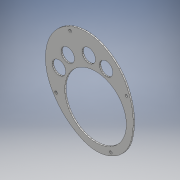
# Autodesk Inventor part: Mano-licar
Saved by Autodesk Inventor 2018 (Build 220112000, 112)
## iProperties
Created: 2019-01-30
Part Number: Mano-licar
Material: Generic
Document SubType Name: Modeling
Designer: Estudiante
Density: 1 g/cm^3
Appearance: Default
Author: Estudiante
Autodesk Inventor part; units mm, degrees
ref_plane "YZ Plane" through (0, 0, 0) normal (1, 0, 0) x (0, 1, 0)
ref_plane "XZ Plane" through (0, 0, 0) normal (0, 1, 0) x (-1, 0, 0)
ref_plane "XY Plane" through (0, 0, 0) normal (0, 0, 1) x (1, 0, 0)
sketch "Sketch1" plane through (0, 0, 0) normal (0, 1, 0) x (-1, 0, 0)
  line L0 (39.5804, 21.3013) -> (36.969, 22.6578)
  line L1 (51.1808, 16.6745) -> (52.2099, 17.5662)
  line L2 (53.4414, 18.1472) -> (52.2099, 17.5662)
  line L3 (54.784, 18.3744) -> (53.4414, 18.1472)
  line L4 (56.1381, 18.231) -> (54.784, 18.3744)
  line L5 (57.4032, 17.7275) -> (56.1381, 18.231)
  line L6 (58.4857, 16.9014) -> (57.4032, 17.7275)
  line L7 (59.3051, 15.8139) -> (58.4857, 16.9014)
  line L8 (59.8007, 14.5456) -> (59.3051, 15.8139)
  line L9 (59.9357, 13.1907) -> (59.8007, 14.5456)
  line L10 (59.7002, 11.8495) -> (59.9357, 13.1907)
  line L11 (59.1116, 10.6216) -> (59.7002, 11.8495)
  line L12 (58.2135, 9.5981) -> (59.1116, 10.6216)
  line L13 (57.0726, 8.8548) -> (58.2135, 9.5981)
  line L14 (55.7735, 8.4469) -> (57.0726, 8.8548)
  line L15 (54.4125, 8.4047) -> (55.7735, 8.4469)
  line L16 (53.0905, 8.7311) -> (54.4125, 8.4047)
  line L17 (51.9057, 9.4022) -> (53.0905, 8.7311)
  line L18 (50.9458, 10.368) -> (51.9057, 9.4022)
  line L19 (50.2822, 11.557) -> (50.9458, 10.368)
  line L20 (49.9639, 12.8809) -> (50.2822, 11.557)
  line L21 (50.0146, 14.2417) -> (49.9639, 12.8809)
  line L22 (50.4305, 15.5382) -> (50.0146, 14.2417)
  line L23 (51.1808, 16.6745) -> (50.4305, 15.5382)
  line L24 (59.8717, 33.0327) -> (61.5031, 30.232)
  line L25 (57.9468, 35.6404) -> (59.8717, 33.0327)
  line L26 (55.751, 38.0245) -> (57.9468, 35.6404)
  line L27 (53.3101, 40.157) -> (55.751, 38.0245)
  line L28 (50.6528, 42.0128) -> (53.3101, 40.157)
  line L29 (47.8103, 43.5703) -> (50.6528, 42.0128)
  line L30 (44.816, 44.8109) -> (47.8103, 43.5703)
  line L31 (41.705, 45.7203) -> (44.816, 44.8109)
  line L32 (38.5138, 46.2877) -> (41.705, 45.7203)
  line L33 (35.28, 46.5065) -> (38.5138, 46.2877)
  line L34 (32.0415, 46.374) -> (35.28, 46.5065)
  line L35 (28.8364, 45.8919) -> (32.0415, 46.374)
  line L36 (25.7022, 45.0658) -> (28.8364, 45.8919)
  line L37 (25.7022, 45.0658) -> (22.2386, 43.6878)
  line L38 (18.9322, 41.9665) -> (22.2386, 43.6878)
  line L39 (15.8169, 39.9196) -> (18.9322, 41.9665)
  line L40 (12.9246, 37.568) -> (15.8169, 39.9196)
  line L41 (10.285, 34.9359) -> (12.9246, 37.568)
  line L42 (7.9252, 32.0504) -> (10.285, 34.9359)
  line L43 (5.8694, 28.9409) -> (7.9252, 32.0504)
  line L44 (4.1387, 25.6393) -> (5.8694, 28.9409)
  line L45 (2.7509, 22.1797) -> (4.1387, 25.6393)
  line L46 (2.7509, 22.1797) -> (1.5483, 18.5508)
  line L47 (0.6396, 14.8374) -> (1.5483, 18.5508)
  line L48 (0.0306, 11.0633) -> (0.6396, 14.8374)
  line L49 (-0.275, 7.2526) -> (0.0306, 11.0633)
  line L50 (-0.275, 3.4296) -> (-0.275, 7.2526)
  line L51 (0.0306, -0.3811) -> (-0.275, 3.4296)
  line L52 (0.6396, -4.1552) -> (0.0306, -0.3811)
  line L53 (1.5483, -7.8686) -> (0.6396, -4.1552)
  line L54 (1.5483, -7.8686) -> (2.5978, -10.8174)
  line L55 (4.0034, -13.6141) -> (2.5978, -10.8174)
  line L56 (5.7437, -16.2157) -> (4.0034, -13.6141)
  line L57 (7.7921, -18.5824) -> (5.7437, -16.2157)
  line L58 (10.117, -20.678) -> (7.7921, -18.5824)
  line L59 (12.6831, -22.4704) -> (10.117, -20.678)
  line L60 (15.4508, -23.9321) -> (12.6831, -22.4704)
  line L61 (15.4508, -23.9321) -> (18.3237, -25.1744)
  line L62 (21.3281, -26.0524) -> (18.3237, -25.1744)
  line L63 (24.4179, -26.5526) -> (21.3281, -26.0524)
  line L64 (27.5458, -26.6672) -> (24.4179, -26.5526)
  line L65 (30.664, -26.3947) -> (27.5458, -26.6672)
  line L66 (33.7246, -25.7391) -> (30.664, -26.3947)
  line L67 (36.6808, -24.7105) -> (33.7246, -25.7391)
  line L68 (36.6808, -24.7105) -> (40.1448, -23.0933)
  line L69 (43.4686, -21.2046) -> (40.1448, -23.0933)
  line L70 (46.6308, -19.0562) -> (43.4686, -21.2046)
  line L71 (49.6112, -16.662) -> (46.6308, -19.0562)
  line L72 (52.3907, -14.0373) -> (49.6112, -16.662)
  line L73 (54.9516, -11.1989) -> (52.3907, -14.0373)
  line L74 (57.2775, -8.1648) -> (54.9516, -11.1989)
  line L75 (59.3535, -4.9547) -> (57.2775, -8.1648)
  line L76 (59.3535, -4.9547) -> (61.1815, -1.706)
  line L77 (62.6715, 1.7109) -> (61.1815, -1.706)
  line L78 (63.8082, 5.261) -> (62.6715, 1.7109)
  line L79 (64.5799, 8.9078) -> (63.8082, 5.261)
  line L80 (64.9788, 12.6141) -> (64.5799, 8.9078)
  line L81 (65.0008, 16.3416) -> (64.9788, 12.6141)
  line L82 (64.6455, 20.0523) -> (65.0008, 16.3416)
  line L83 (63.9167, 23.708) -> (64.6455, 20.0523)
  line L84 (62.8219, 27.2712) -> (63.9167, 23.708)
  line L85 (61.5031, 30.232) -> (62.8219, 27.2712)
  line L86 (49.2473, 19.8424) -> (50.5464, 20.2503)
  line L87 (47.8862, 19.8002) -> (49.2473, 19.8424)
  line L88 (46.5643, 20.1267) -> (47.8862, 19.8002)
  line L89 (45.3795, 20.7977) -> (46.5643, 20.1267)
  line L90 (44.4196, 21.7635) -> (45.3795, 20.7977)
  line L91 (43.7559, 22.9525) -> (44.4196, 21.7635)
  line L92 (43.4376, 24.2764) -> (43.7559, 22.9525)
  line L93 (43.4883, 25.6372) -> (43.4376, 24.2764)
  line L94 (43.9043, 26.9337) -> (43.4883, 25.6372)
  line L95 (44.6546, 28.07) -> (43.9043, 26.9337)
  line L96 (44.6546, 28.07) -> (45.6837, 28.9617)
  line L97 (46.9152, 29.5427) -> (45.6837, 28.9617)
  line L98 (48.2578, 29.7699) -> (46.9152, 29.5427)
  line L99 (49.6118, 29.6265) -> (48.2578, 29.7699)
  line L100 (50.877, 29.123) -> (49.6118, 29.6265)
  line L101 (51.9594, 28.2969) -> (50.877, 29.123)
  line L102 (52.7788, 27.2094) -> (51.9594, 28.2969)
  line L103 (53.2745, 25.9411) -> (52.7788, 27.2094)
  line L104 (53.4095, 24.5862) -> (53.2745, 25.9411)
  line L105 (53.174, 23.245) -> (53.4095, 24.5862)
  line L106 (52.5854, 22.0172) -> (53.174, 23.245)
  line L107 (51.6873, 20.9936) -> (52.5854, 22.0172)
  line L108 (50.5464, 20.2503) -> (51.6873, 20.9936)
  line L109 (45.6686, 41.0487) -> (45.8931, 40.5319)
  line L110 (45.6686, 41.0487) -> (45.7592, 41.6049)
  line L111 (45.7592, 41.6049) -> (46.136, 42.0238)
  line L112 (46.136, 42.0238) -> (46.6795, 42.1724)
  line L113 (47.2171, 42.0036) -> (46.6795, 42.1724)
  line L114 (47.5781, 41.571) -> (47.2171, 42.0036)
  line L115 (47.6479, 41.0119) -> (47.5781, 41.571)
  line L116 (47.4044, 40.5038) -> (47.6479, 41.0119)
  line L117 (46.9247, 40.208) -> (47.4044, 40.5038)
  line L118 (46.3614, 40.2185) -> (46.9247, 40.208)
  line L119 (45.8931, 40.5319) -> (46.3614, 40.2185)
  line L120 (36.9503, 29.5123) -> (37.539, 30.7402)
  line L121 (36.0523, 28.4888) -> (36.9503, 29.5123)
  line L122 (34.9114, 27.7455) -> (36.0523, 28.4888)
  line L123 (33.6122, 27.3376) -> (34.9114, 27.7455)
  line L124 (32.2512, 27.2953) -> (33.6122, 27.3376)
  line L125 (30.9293, 27.6218) -> (32.2512, 27.2953)
  line L126 (29.7444, 28.2929) -> (30.9293, 27.6218)
  line L127 (28.7846, 29.2587) -> (29.7444, 28.2929)
  line L128 (28.1209, 30.4477) -> (28.7846, 29.2587)
  line L129 (27.8026, 31.7716) -> (28.1209, 30.4477)
  line L130 (27.8533, 33.1323) -> (27.8026, 31.7716)
  line L131 (28.2692, 34.4289) -> (27.8533, 33.1323)
  line L132 (29.0196, 35.5652) -> (28.2692, 34.4289)
  line L133 (29.0196, 35.5652) -> (30.0486, 36.4569)
  line L134 (31.2801, 37.0379) -> (30.0486, 36.4569)
  line L135 (32.6227, 37.2651) -> (31.2801, 37.0379)
  line L136 (33.9768, 37.1217) -> (32.6227, 37.2651)
  line L137 (35.242, 36.6182) -> (33.9768, 37.1217)
  line L138 (36.3244, 35.7921) -> (35.242, 36.6182)
  line L139 (37.1438, 34.7046) -> (36.3244, 35.7921)
  line L140 (37.6394, 33.4363) -> (37.1438, 34.7046)
  line L141 (37.7745, 32.0813) -> (37.6394, 33.4363)
  line L142 (37.539, 30.7402) -> (37.7745, 32.0813)
  line L143 (19.8181, -19.9229) -> (22.6407, -20.7551)
  line L144 (17.1252, -18.7365) -> (19.8181, -19.9229)
  line L145 (14.6061, -17.2156) -> (17.1252, -18.7365)
  line L146 (12.3022, -15.385) -> (14.6061, -17.2156)
  line L147 (10.2513, -13.2748) -> (12.3022, -15.385)
  line L148 (8.4871, -10.9196) -> (10.2513, -13.2748)
  line L149 (7.0385, -8.3582) -> (8.4871, -10.9196)
  line L150 (5.9294, -5.6326) -> (7.0385, -8.3582)
  line L151 (5.1779, -2.7875) -> (5.9294, -5.6326)
  line L152 (4.7964, 0.1303) -> (5.1779, -2.7875)
  line L153 (4.7912, 3.073) -> (4.7964, 0.1303)
  line L154 (5.1623, 5.9921) -> (4.7912, 3.073)
  line L155 (5.9036, 8.8399) -> (5.1623, 5.9921)
  line L156 (5.9036, 8.8399) -> (7.003, 11.5694)
  line L157 (7.003, 11.5694) -> (8.4425, 14.136)
  line L158 (8.4425, 14.136) -> (10.1983, 16.4974)
  line L159 (12.2417, 18.6149) -> (10.1983, 16.4974)
  line L160 (14.5391, 20.4537) -> (12.2417, 18.6149)
  line L161 (17.0527, 21.9836) -> (14.5391, 20.4537)
  line L162 (19.7414, 23.1795) -> (17.0527, 21.9836)
  line L163 (22.561, 24.0218) -> (19.7414, 23.1795)
  line L164 (25.465, 24.4966) -> (22.561, 24.0218)
  line L165 (28.406, 24.5962) -> (25.465, 24.4966)
  line L166 (31.3356, 24.3188) -> (28.406, 24.5962)
  line L167 (34.2056, 23.6692) -> (31.3356, 24.3188)
  line L168 (36.969, 22.6578) -> (34.2056, 23.6692)
  line L169 (39.5804, 21.3013) -> (36.969, 22.6578)
  line L170 (41.9968, 19.6221) -> (39.5804, 21.3013)
  line L171 (44.1787, 17.6476) -> (41.9968, 19.6221)
  line L172 (46.0902, 15.4104) -> (44.1787, 17.6476)
  line L173 (47.6999, 12.947) -> (46.0902, 15.4104)
  line L174 (48.9814, 10.2981) -> (47.6999, 12.947)
  line L175 (49.9137, 7.507) -> (48.9814, 10.2981)
  line L176 (50.4813, 4.6196) -> (49.9137, 7.507)
  line L177 (50.6751, 1.6833) -> (50.4813, 4.6196)
  line L178 (50.4918, -1.2536) -> (50.6751, 1.6833)
  line L179 (49.9344, -4.143) -> (50.4918, -1.2536)
  line L180 (49.0121, -6.9374) -> (49.9344, -4.143)
  line L181 (47.7401, -9.5909) -> (49.0121, -6.9374)
  line L182 (46.1391, -12.0599) -> (47.7401, -9.5909)
  line L183 (44.2356, -14.304) -> (46.1391, -12.0599)
  line L184 (42.0608, -16.2862) -> (44.2356, -14.304)
  line L185 (39.6503, -17.9741) -> (42.0608, -16.2862)
  line L186 (37.0438, -19.3398) -> (39.6503, -17.9741)
  line L187 (34.284, -20.361) -> (37.0438, -19.3398)
  line L188 (31.4163, -21.0209) -> (34.284, -20.361)
  line L189 (28.4877, -21.3087) -> (31.4163, -21.0209)
  line L190 (25.5464, -21.2196) -> (28.4877, -21.3087)
  line L191 (22.6407, -20.7551) -> (25.5464, -21.2196)
  line L192 (15.8354, -21.1838) -> (16.3789, -21.0352)
  line L193 (16.9165, -21.204) -> (16.3789, -21.0352)
  line L194 (17.2775, -21.6366) -> (16.9165, -21.204)
  line L195 (17.3472, -22.1957) -> (17.2775, -21.6366)
  line L196 (17.1037, -22.7038) -> (17.3472, -22.1957)
  line L197 (16.6241, -22.9996) -> (17.1037, -22.7038)
  line L198 (16.0607, -22.9891) -> (16.6241, -22.9996)
  line L199 (15.5924, -22.6757) -> (16.0607, -22.9891)
  line L200 (15.3679, -22.1589) -> (15.5924, -22.6757)
  line L201 (15.3679, -22.1589) -> (15.4585, -21.6027)
  line L202 (15.4585, -21.6027) -> (15.8354, -21.1838)
  line L203 (3.7713, 20.5816) -> (4.1481, 21.0005)
  line L204 (4.1481, 21.0005) -> (4.6916, 21.1491)
  line L205 (5.2292, 20.9803) -> (4.6916, 21.1491)
  line L206 (5.5902, 20.5477) -> (5.2292, 20.9803)
  line L207 (5.66, 19.9886) -> (5.5902, 20.5477)
  line L208 (5.4164, 19.4805) -> (5.66, 19.9886)
  line L209 (4.9368, 19.1847) -> (5.4164, 19.4805)
  line L210 (4.3735, 19.1952) -> (4.9368, 19.1847)
  line L211 (3.9052, 19.5086) -> (4.3735, 19.1952)
  line L212 (3.6807, 20.0254) -> (3.9052, 19.5086)
  line L213 (3.6807, 20.0254) -> (3.7713, 20.5816)
  line L214 (57.6736, -3.0517) -> (57.136, -2.8829)
  line L215 (58.0346, -3.4843) -> (57.6736, -3.0517)
  line L216 (58.1044, -4.0434) -> (58.0346, -3.4843)
  line L217 (57.8608, -4.5515) -> (58.1044, -4.0434)
  line L218 (57.3812, -4.8473) -> (57.8608, -4.5515)
  line L219 (56.8178, -4.8368) -> (57.3812, -4.8473)
  line L220 (56.3496, -4.5234) -> (56.8178, -4.8368)
  line L221 (56.1251, -4.0066) -> (56.3496, -4.5234)
  line L222 (56.1251, -4.0066) -> (56.2156, -3.4504)
  line L223 (56.2156, -3.4504) -> (56.5925, -3.0315)
  line L224 (56.5925, -3.0315) -> (57.136, -2.8829)
  line L225 (24.5678, 28.6914) -> (24.8033, 30.0326)
  line L226 (23.9791, 27.4636) -> (24.5678, 28.6914)
  line L227 (23.0811, 26.44) -> (23.9791, 27.4636)
  line L228 (21.9402, 25.6968) -> (23.0811, 26.44)
  line L229 (20.641, 25.2889) -> (21.9402, 25.6968)
  line L230 (19.28, 25.2466) -> (20.641, 25.2889)
  line L231 (17.9581, 25.5731) -> (19.28, 25.2466)
  line L232 (16.7732, 26.2441) -> (17.9581, 25.5731)
  line L233 (15.8134, 27.2099) -> (16.7732, 26.2441)
  line L234 (15.1497, 28.3989) -> (15.8134, 27.2099)
  line L235 (14.8314, 29.7229) -> (15.1497, 28.3989)
  line L236 (14.8821, 31.0836) -> (14.8314, 29.7229)
  line L237 (15.298, 32.3802) -> (14.8821, 31.0836)
  line L238 (16.0484, 33.5164) -> (15.298, 32.3802)
  line L239 (16.0484, 33.5164) -> (17.0775, 34.4081)
  line L240 (18.3089, 34.9891) -> (17.0775, 34.4081)
  line L241 (19.6515, 35.2164) -> (18.3089, 34.9891)
  line L242 (21.0056, 35.0729) -> (19.6515, 35.2164)
  line L243 (22.2708, 34.5695) -> (21.0056, 35.0729)
  line L244 (23.3532, 33.7433) -> (22.2708, 34.5695)
  line L245 (24.1726, 32.6558) -> (23.3532, 33.7433)
  line L246 (24.6682, 31.3875) -> (24.1726, 32.6558)
  line L247 (24.8033, 30.0326) -> (24.6682, 31.3875)
  point P0 (0, 0)
  constraints: 496 end point
extrude "Extrusion1" add sketch "Sketch1" along normal blind 1
body "Solid1"
